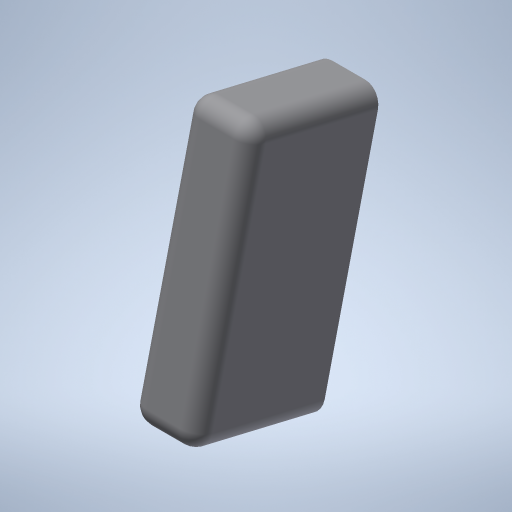
# Autodesk Inventor part: caja de los actuadores
Saved by Autodesk Inventor 2023 (Build 270158000, 158)
## iProperties
Created: 2022-10-17
Part Number: caja de los actuadores
Material: Generic
Document SubType Name: Modeling
Designer: Xiaba
Density: 1 g/cm^3
Appearance: Default
Author: Xiaba
Autodesk Inventor part; units mm, degrees
ref_plane "YZ Plane" through (0, 0, 0) normal (1, 0, 0) x (0, 1, 0)
ref_plane "XZ Plane" through (0, 0, 0) normal (0, 1, 0) x (-1, 0, 0)
sketch "Sketch1" plane through (0, 0, 0) normal (1, 0, 0) x (0, 1, 0)
  line L0 (0, 0) -> (67.821, 0)
  line L1 (67.821, 0) -> (67.821, -16.094)
  line L2 (67.821, -16.094) -> (0, -16.094)
  line L3 (0, -16.094) -> (0, 0)
  line L4 (67.821, -16.094) -> (0, 0)
  dimension "d0" = 67.821
  dimension "d1" = 16.094
  constraints: 10 end point, 2 parallel, 1 horizontal, 1 perpendicular
  measures "d0" distance of L1.end L2.end
  measures "d1" distance of L0.end L1.end
ref_plane "Work Plane1" through (0, 0, 0) normal (0, 0.2308893, 0.97298) x (1, 0, 0)
sketch "Sketch4" plane through (0, 0, 0) normal (0, 0.2308893, 0.97298) x (1, 0, 0)
  line L0 (0, 0) -> (-10, 0)
  line L1 (-10, 0) -> (-10, -40)
  line L2 (-10, -40) -> (0, -40)
  line L3 (0, -40) -> (0, 0)
  dimension "d16" = 40
  dimension "d17" = 10
  constraints: 8 end point, 2 parallel, 1 horizontal, 1 perpendicular
  measures "d16" distance of L0.end L1.end
  measures "d17" distance of L1.end L2.end
extrude "Extrusion4" add sketch "Sketch4" along normal blind 20
fillet "Fillet3" radius 2.5 8 edges at (0, -14.8418, 24.0774) (-10, -14.8418, 24.0774) (-5, 4.6178, 19.4596) (-10, 2.3089, 9.7298) (0, 2.3089, 9.7298) (0, -36.6103, 18.9654) (-5, -34.3014, 28.6952) (-10, -36.6103, 18.9654)
shell "Shell2" thickness 1 removed faces 0
sketch "Sketch5" plane through (-7.5, -38.9192, 9.2356) normal (0, -0.97298, 0.2308893) x (1, 0, 0)
  line L0 (0, 0) -> (0, 17.5) projected
  line L1 (0, 0) -> (5, 0) projected
  line L2 (5, 17.5) -> (5, 0) projected
  line L3 (0, 17.5) -> (5, 17.5) projected
  circle A0 centre (2.5, 14.5) radius 1.5
  point P0 (7.5, 0)
  point P1 (2.5, 17.5)
  dimension "d22" = 3
  dimension "d23" = 3
  constraints: 1 centre point, 1 midpoint
  measures "d22" diameter of A0
  measures "d23" distance of point (2.5, 17.5) A0.centre
extrude "Extrusion5" cut sketch "Sketch5" against normal blind 2 contours A0
fillet "Fillet4" radius 0.5 2 edges at (-6.5, -34.5983, 23.1129) (-6.5, -35.5713, 23.3438)
sketch "Sketch6" plane through (0, -36.4868, 8.6583) normal (1, 0, 0) x (0, -0.2308893, -0.97298)
  line L0 (-17.5, 35) -> (0, 35) projected
  line L1 (-17.5, 0) -> (-17.5, 35) projected
  line L2 (0, 0) -> (-17.5, 0) projected
  line L3 (0, 0) -> (0, 35) projected
  point P0 (0, 37.5)
  dimension "d27" = 35
  dimension "d28" = 17.5
  measures "d27" distance of L1.start L0.start
  measures "d28" distance of L0.start L0.end
sketch "Sketch7" plane through (-10, -36.4868, 8.6583) normal (-1, 0, 0) x (0, 0.2308893, 0.97298)
  line L0 (0, -2.5) -> (17.5, -2.5) projected
  line L1 (20, 0) -> (20, 35) projected
  line L2 (20, -2.5) -> (6.9383, -2.5)
  line L3 (7.5, 6.273) -> (20, 6.273)
  line L4 (20, 6.273) -> (20, -2.5)
  line L5 (0, -2.5) -> (20, -2.5)
  line L6 (12.5, -2.5) -> (16.5, -2.5) projected
  line L7 (20, 6.273) -> (20, -2.5)
  line L8 (20, -2.5) -> (20, 16.6364)
  line L9 (20, 35) -> (20, 0) projected
  line L10 (7.5, 6.273) -> (7.5, -2.5)
  circle A0 centre (7.5, 6.273) radius 0.75
  point P0 (0, 37.5)
  dimension "d29" = 12.5
  dimension "d30" = 8.773
  dimension "d31" = 1.5
  constraints: 14 end point, 2 collinear, 2 point on line, 1 centre point, 1 coincident, 1 horizontal, 1 parallel, 1 perpendicular
  measures "d29" distance of L3.start L3.end
  measures "d30" distance of L3.start L10.end
  measures "d31" diameter of A0
extrude "Extrusion6" add sketch "Sketch7" against normal blind 10 contours A0 L3 L10 | L10 L3 A0
body "Solid2"
